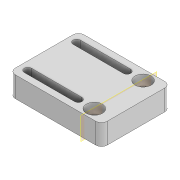
# Autodesk Inventor part: intake motor mount to xrail fixed position
Saved by Autodesk Inventor 2020 (Build 240168000, 168)
## iProperties
Created: 2020-01-10
Part Number: intake motor mount to xrail fixed position
Material: Generic
Document SubType Name: Modeling
Designer: ball
Density: 1 g/cm^3
Appearance: Default
Author: ball
Autodesk Inventor part; units mm, degrees
ref_plane "XZ Plane" through (0, 0, 0) normal (0, 1, 0) x (-1, 0, 0)
ref_plane "XY Plane" through (0, 0, 0) normal (0, 0, 1) x (1, 0, 0)
sketch "Sketch1" plane through (0, 0, 0) normal (0, 1, 0) x (-1, 0, 0)
  line L0 (-9.525, 19.05) -> (41.275, 19.05)
  line L1 (41.275, 19.05) -> (41.275, -19.05)
  line L2 (41.275, -19.05) -> (-9.525, -19.05)
  line L3 (-9.525, -19.05) -> (-9.525, 19.05)
  point P0 (0, 0)
  dimension "d0" = 50.8
  dimension "d1" = 38.1
  dimension "d3" = 9.525
  dimension "d4" = 19.05
  constraints: 8 end point, 2 parallel, 1 horizontal, 1 perpendicular
  measures "d0" distance of L1.end L2.end
  measures "d1" distance of L0.end L1.end
  measures "d3" distance from line of L3 point (0, 0)
  measures "d4" distance from line of L0 point (0, 0)
extrude "Extrusion1" add sketch "Sketch1" along normal blind 11.43
sketch "Sketch2" plane through (0, 11.43, 0) normal (0, 1, 0) x (1, 0, 0)
  line L0 (9.525, -19.05) -> (9.525, 19.05) projected
  point P0 (0, 0)
  point P1 (0, -13.4747)
  point P2 (0, 13.4747)
  dimension "d7" = 26.9494
  dimension "d9" = 9.525
  dimension "d10" = 9.525
  dimension "d11" = 13.4747
  measures "d7" distance of point (0, 13.475) point (0, -13.475)
  measures "d9" distance from line of L0 point (0, -13.475)
  measures "d10" distance from line of L0 point (0, 13.475)
  measures "d11" distance of point (0, -13.475) point (0, 0)
hole "Hole1" at (0, 11.43, 13.4747) at (0, 11.43, -13.4747) direction (0, -1, 0) diameter 4.064 end through all counterbore diameter 8.89 counterbore depth 5.9436
sketch "Sketch3" plane through (0, 0, 0) normal (0, -1, 0) x (1, 0, 0)
  circle A0 centre (0, -13.4747) radius 2.032 projected
  circle A1 centre (0, 13.4747) radius 2.032 projected
  line L0 (-41.275, -19.05) -> (-41.275, 19.05) projected
  line L1 (-36.703, -13.4747) -> (-8.89, -13.4747) construction
  line L2 (-36.703, -15.5067) -> (-8.89, -15.5067)
  line L3 (-8.89, -11.4427) -> (-36.703, -11.4427)
  arc A2 (-36.703, -11.4427) -> (-36.703, -15.5067) centre (-36.703, -13.4747) ccw
  arc A3 (-8.89, -15.5067) -> (-8.89, -11.4427) centre (-8.89, -13.4747) ccw
  line L4 (-36.703, 13.4747) -> (-8.89, 13.4747) construction
  line L5 (-36.703, 11.4427) -> (-8.89, 11.4427)
  line L6 (-8.89, 15.5067) -> (-36.703, 15.5067)
  arc A4 (-36.703, 15.5067) -> (-36.703, 11.4427) centre (-36.703, 13.4747) ccw
  arc A5 (-8.89, 11.4427) -> (-8.89, 15.5067) centre (-8.89, 13.4747) ccw
  point P0 (0, 0)
  point P1 (-22.7965, -13.4747)
  point P2 (-22.7965, 13.4747)
  dimension "d19" = 26.9494
  dimension "d20" = 13.4747
  dimension "d21" = 8.89
  dimension "d22" = 8.89
  dimension "d23" = 4.572
  dimension "d24" = 4.572
  dimension "d25" = 4.064
  dimension "d26" = 4.064
  constraints: 16 end point, 8 point on circle, 8 tangent, 4 centre point, 3 parallel, 2 midpoint, 1 horizontal
  measures "d19" distance of L4.end L1.end
  measures "d20" vertical distance of point (0, 0) L1.end
  measures "d21" distance of A0.centre L1.end
  measures "d22" distance of A1.centre L4.end
  measures "d23" distance from line of L0 L1.start
  measures "d24" distance from line of L0 L4.start
  measures "d25" diameter of A3
  measures "d26" diameter of A5
extrude "Extrusion2" cut sketch "Sketch3" against normal through all contours A2 L3 A3 L2 | A4 L6 A5 L5
sketch "Sketch4" plane through (0, 0, 0) normal (0, -1, 0) x (1, 0, 0)
  arc A0 (-36.703, 15.5067) -> (-36.703, 11.4427) centre (-36.703, 13.4747) ccw projected
  arc A1 (-8.89, 11.4427) -> (-8.89, 15.5067) centre (-8.89, 13.4747) ccw projected
  line L0 (-36.703, 13.4747) -> (-8.89, 13.4747) construction
  line L1 (-36.703, 9.0297) -> (-8.89, 9.0297)
  line L2 (-8.89, 17.9197) -> (-36.703, 17.9197)
  arc A2 (-36.703, 17.9197) -> (-36.703, 9.0297) centre (-36.703, 13.4747) ccw
  arc A3 (-8.89, 9.0297) -> (-8.89, 17.9197) centre (-8.89, 13.4747) ccw
  arc A4 (-8.89, -15.5067) -> (-8.89, -11.4427) centre (-8.89, -13.4747) ccw projected
  arc A5 (-36.703, -11.4427) -> (-36.703, -15.5067) centre (-36.703, -13.4747) ccw projected
  line L3 (-8.89, -13.4747) -> (-36.703, -13.4747) construction
  line L4 (-8.89, -9.0297) -> (-36.703, -9.0297)
  line L5 (-36.703, -17.9197) -> (-8.89, -17.9197)
  arc A6 (-8.89, -17.9197) -> (-8.89, -9.0297) centre (-8.89, -13.4747) ccw
  arc A7 (-36.703, -9.0297) -> (-36.703, -17.9197) centre (-36.703, -13.4747) ccw
  point P0 (0, 0)
  point P1 (-22.7965, 13.4747)
  point P2 (-22.7965, -13.4747)
  dimension "d29" = 8.89
  dimension "d30" = 8.89
  constraints: 16 end point, 8 point on circle, 8 tangent, 4 centre point, 3 parallel, 2 midpoint, 1 horizontal
  measures "d29" diameter of A3
  measures "d30" diameter of A7
extrude "Extrusion3" cut sketch "Sketch4" against normal blind 6.35
fillet "Fillet1" radius 3.175 4 edges at (9.525, 5.715, 19.05) (9.525, 5.715, -19.05) (-41.275, 5.715, 19.05) (-41.275, 5.715, -19.05)
equation "\"d4\" = 0.5 * d1"
equation "\"d9\" = d3"
equation "\"d10\" = d9"
equation "\"d11\" = 0.5 * d7"
equation "\"d20\" = 0.5 * d19"
equation "\"d22\" = d21"
equation "\"d24\" = d23"
equation "\"d26\" = d25"
equation "\"d30\" = d29"
body "Solid1"
